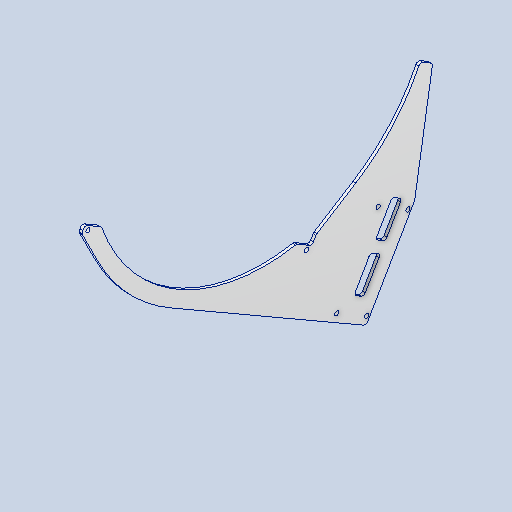
# Autodesk Inventor part: belt_liner_v2_Plate_6
Saved by Autodesk Inventor 2025.2 (Build 292293000, 293)
## iProperties
Created: 2025-01-06
Part Number: belt_liner_v2_Plate_6
Material: アルミニウム 6061
Document SubType Name: Modeling
Designer: haruy
Density: 2.7 g/cm^3
Appearance: アルミニウム - フラット
Author: haruy
Autodesk Inventor part; units mm, degrees
ref_plane "YZ Plane" through (0, 0, 0) normal (1, 0, 0) x (0, 1, 0)
ref_plane "XZ Plane" through (0, 0, 0) normal (0, 1, 0) x (-1, 0, 0)
ref_plane "XY Plane" through (0, 0, 0) normal (0, 0, 1) x (1, 0, 0)
derived "belt_liner_v2_Sketch_Base.ipt"
sketch "スケッチ1" plane through (300, 0, 0) normal (1, 0, 0) x (0, 1, 0)
  circle A0 centre (0, 0) radius 22.36
  circle A1 centre (742.400277, -428.625) radius 23.875 construction
  line L0 (0, 0) -> (0, -985.832038)
  line L1 (4.693429, 56.249257) -> (12.193429, 69.239638)
  line L2 (12.193429, 69.239638) -> (479.847147, -200.760362)
  line L3 (479.847147, -200.760362) -> (472.347147, -213.750743)
  line L4 (472.347147, -213.750743) -> (4.693429, 56.249257)
  line L5 (0, 0) -> (742.400277, -428.625)
  line L6 (-43.599071, -27.395807) -> (-51.099071, -40.386188)
  line L7 (-51.099071, -40.386188) -> (711.003284, -480.386188)
  line L8 (711.003284, -480.386188) -> (718.503284, -467.395807)
  line L9 (718.503284, -467.395807) -> (-43.599071, -27.395807)
  line L10 (-64.855825, 113.724045) -> (-64.855825, 113.724045)
  line L11 (4.693429, 56.249257) -> (0.351336, 58.756166)
  line L12 (0.351336, 58.756166) -> (-2.148664, 54.426038)
  line L13 (-2.148664, 54.426038) -> (2.193429, 51.91913)
  line L14 (2.193429, 51.91913) -> (4.693429, 56.249257)
  line L15 (472.347147, -213.750743) -> (374.172186, -157.069403)
  line L16 (0, -985.832038) -> (0, 0)
  circle A2 centre (0, 0) radius 12.5
  circle A3 centre (0, 0) radius 15
  line L17 (0, 0) -> (0, 0)
  circle A4 centre (0, 0) radius 24.06 construction
  line L18 (0, 0) -> (0, 0)
  line L19 (0, 0) -> (0, 0)
  line L20 (-43.599071, -27.395807) -> (-41.099071, -23.065679)
  line L21 (-41.099071, -23.065679) -> (28.918099, -63.490111)
  line L22 (32.480276, -71.320238) -> (-43.599071, -27.395807)
  line L23 (85.805588, 26.739638) -> (479.847147, -200.760362)
  line L24 (479.847147, -200.760362) -> (482.597147, -195.997222)
  circle A5 centre (742.400277, -428.625) radius 5
  line L25 (718.503284, -467.395807) -> (692.522522, -452.395807)
  line L26 (692.522522, -452.395807) -> (695.022522, -448.065679)
  line L27 (695.022522, -448.065679) -> (721.003284, -463.065679)
  line L28 (721.003284, -463.065679) -> (718.503284, -467.395807)
  circle A6 centre (738.07015, -426.125) radius 5.1
  line L29 (742.400277, -428.625) -> (511.038915, -295.048455)
  circle A7 centre (759.720785, -438.625) radius 5.1
  line L30 (740.62015, -421.70827) -> (762.270785, -434.20827)
  line L31 (735.52015, -430.54173) -> (757.170785, -443.04173)
  circle A8 centre (742.400277, -428.625) radius 22.175 construction
  line L32 (792.376136, -398.519566) -> (776.376136, -426.232379)
  line L33 (776.376136, -426.232379) -> (785.03639, -431.232379)
  line L34 (785.03639, -431.232379) -> (801.03639, -403.519566)
  line L35 (801.03639, -403.519566) -> (792.376136, -398.519566)
  circle A9 centre (738.07015, -426.125) radius 10.1 construction
  circle A10 centre (759.720785, -438.625) radius 10.1 construction
  line L36 (743.12015, -417.378143) -> (764.770785, -429.878143) construction
  line L37 (733.02015, -434.871857) -> (754.670785, -447.371857) construction
  line L38 (743.12015, -417.378143) -> (732.666299, -411.34261) construction
  line L39 (729.323294, -421.075) -> (734.373294, -412.328143) construction
  line L40 (764.770785, -429.878143) -> (773.093818, -434.683448) construction
  line L41 (773.093818, -434.683448) -> (773.43104, -434.878143)
  line L42 (0.351336, 58.756166) -> (-2.148664, 54.426038)
  line L43 (-2.148664, 54.426038) -> (100.487312, -4.83087)
  line L44 (100.487312, -4.83087) -> (102.987312, -0.500743)
  line L45 (102.987312, -0.500743) -> (0.351336, 58.756166)
  line L46 (-51.099071, -40.386188) -> (-51.099071, -619.920903)
  line L47 (754.670785, -447.371857) -> (764.770785, -429.878143)
  line L48 (764.770785, -429.878143) -> (773.43104, -434.878143)
  line L49 (773.43104, -434.878143) -> (763.33104, -452.371857)
  line L50 (763.33104, -452.371857) -> (754.670785, -447.371857) construction
  line L51 (479.847147, -200.760362) -> (472.347147, -213.750743)
  line L52 (472.347147, -213.750743) -> (896.699557, -458.750721)
  line L53 (896.699557, -458.750721) -> (904.199557, -445.76034)
  line L54 (904.199557, -445.76034) -> (479.847147, -200.760362)
  line L55 (-12.152186, -2.928204) -> (-38.10869, -47.886188)
  line L56 (-12.152186, -2.928204) -> (25.18381, 61.739638)
  circle A11 centre (38.084445, 34.084194) radius 1.5
  circle A12 centre (59.73508, 21.584194) radius 1.5
  circle A13 centre (711.09303, -460.230743) radius 1.5
  circle A14 centre (0, 0) radius 60
  line L57 (54.694812, -84.145807) -> (57.194812, -79.815679)
  line L58 (100.487312, -4.83087) -> (57.194812, -79.815679)
  circle A15 centre (81.385715, 9.084194) radius 1.5
  circle A16 centre (742.400277, -428.625) radius 6 construction
  circle A17 centre (0, 0) radius 24.06 construction
  circle A18 centre (0, 0) radius 24.06
  circle A19 centre (742.400277, -428.625) radius 24.06
  line L59 (754.430277, -407.788429) -> (12.03, 20.836571)
  circle A20 centre (725.859192, -419.075) radius 4
  circle A21 centre (725.859192, -419.075) radius 1.5
  circle A22 centre (742.400277, -428.625) radius 18.525 construction
  circle A23 centre (748.98688, -417.41667) radius 4
  line L60 (737.43688, -437.421857) -> (742.48688, -428.675)
  circle A24 centre (748.98688, -417.41667) radius 1.5
  line L61 (734.373294, -412.328143) -> (737.823294, -406.352568) construction
  line L62 (737.823294, -406.352568) -> (776.88104, -428.902568)
  line L63 (773.43104, -434.878143) -> (776.88104, -428.902568)
  line L64 (737.823294, -406.352568) -> (723.650341, -415.740187)
  line L65 (720.823294, -435.797432) -> (759.88104, -458.347432)
  line L66 (720.823294, -435.797432) -> (721.866734, -418.829485)
  line L67 (763.33104, -452.371857) -> (759.88104, -458.347432)
  circle A25 centre (735.98688, -439.93333) radius 4
  circle A26 centre (735.98688, -439.93333) radius 1.5
  circle A27 centre (300.529907, 58.653068) radius 120
  line L68 (24.788304, 15.779962) -> (16.12805, 20.779962) construction
  line L69 (896.699557, -458.750721) -> (870.718795, -443.750721)
  line L70 (870.718795, -443.750721) -> (868.218795, -448.080848)
  line L71 (868.218795, -448.080848) -> (894.199557, -463.080848)
  line L72 (894.199557, -463.080848) -> (896.699557, -458.750721)
  circle A28 centre (886.789303, -455.915785) radius 1.5
  line L73 (100.487312, -4.83087) -> (102.987312, -0.500743)
  line L74 (102.987312, -0.500743) -> (112.946604, -6.250743)
  line L75 (112.946604, -6.250743) -> (110.446604, -10.58087)
  line L76 (110.446604, -10.58087) -> (100.487312, -4.83087)
  circle A29 centre (878.129049, -450.915785) radius 1.5
  circle A30 centre (702.432776, -455.230743) radius 1.5
  line L77 (28.918099, -63.490111) -> (57.194812, -79.815679)
  line L78 (479.847147, -200.760362) -> (482.597147, -195.997222)
  line L79 (121.446604, 8.471689) -> (179.903319, -25.278311)
  line L80 (179.903319, -25.278311) -> (182.403319, -20.948184)
  line L81 (182.403319, -20.948184) -> (123.946604, 12.801816)
  line L82 (123.946604, 12.801816) -> (121.446604, 8.471689)
  circle A31 centre (135.905896, 10.515918) radius 4
  circle A32 centre (135.905896, 10.515918) radius 11
  circle A33 centre (161.886659, -4.484082) radius 4
  circle A34 centre (161.886659, -4.484082) radius 11
  line L83 (131.869998, -4.474463) -> (128.369998, -10.536641)
  line L84 (128.369998, -10.536641) -> (147.422557, -21.536641)
  line L85 (147.422557, -21.536641) -> (150.922557, -15.474463)
  line L86 (150.922557, -15.474463) -> (131.869998, -4.474463)
  line L87 (141.396277, -9.974463) -> (137.896277, -16.036641)
  line L88 (157.85076, -19.474463) -> (154.35076, -25.536641)
  line L89 (154.35076, -25.536641) -> (173.403319, -36.536641)
  line L90 (173.403319, -36.536641) -> (176.903319, -30.474463)
  line L91 (176.903319, -30.474463) -> (157.85076, -19.474463)
  line L92 (167.37704, -24.974463) -> (163.87704, -31.036641)
  line L93 (8.443429, 62.744448) -> (900.449557, -452.255531)
  line L94 (170.403319, -41.732794) -> (167.903319, -46.062921)
  line L95 (111.946604, -7.982794) -> (170.403319, -41.732794)
  line L96 (167.903319, -46.062921) -> (109.446604, -12.312921)
  line L97 (109.446604, -12.312921) -> (111.946604, -7.982794)
  circle A35 centre (117.405896, -21.527022) radius 11
  circle A36 centre (117.405896, -21.527022) radius 4
  circle A37 centre (143.386659, -36.527022) radius 11
  circle A38 centre (143.386659, -36.527022) radius 4
  line L98 (140.932176, -2.778311) -> (147.860379, -6.778311)
  line L99 (147.860379, -6.778311) -> (138.360379, -23.232794)
  line L100 (138.360379, -23.232794) -> (131.432176, -19.232794)
  line L101 (131.432176, -19.232794) -> (140.932176, -2.778311)
  line L102 (166.912938, -17.778311) -> (173.841141, -21.778311)
  line L103 (173.841141, -21.778311) -> (164.341141, -38.232794)
  line L104 (164.341141, -38.232794) -> (157.412938, -34.232794)
  line L105 (157.412938, -34.232794) -> (166.912938, -17.778311)
  line L106 (109.446604, -12.312921) -> (96.946604, -33.963556)
  line L107 (96.946604, -33.963556) -> (105.606858, -38.963556)
  line L108 (105.606858, -38.963556) -> (118.106858, -17.312921)
  line L109 (118.106858, -17.312921) -> (109.446604, -12.312921)
  line L110 (109.446604, -12.312921) -> (144.953646, -32.812921)
  line L111 (144.953646, -32.812921) -> (140.953646, -39.741124)
  line L112 (140.953646, -39.741124) -> (105.446604, -19.241124)
  line L113 (105.446604, -19.241124) -> (109.446604, -12.312921)
  line L114 (128.932176, -23.562921) -> (135.860379, -27.562921)
  line L115 (135.860379, -27.562921) -> (134.360379, -30.160997)
  line L116 (134.360379, -30.160997) -> (127.432176, -26.160997)
  line L117 (127.432176, -26.160997) -> (128.932176, -23.562921)
  circle A39 centre (-7.708055, -45.230743) radius 1.25
  circle A40 centre (13.94258, -57.730743) radius 1.25
  circle A41 centre (35.593215, -70.230743) radius 1.25
  circle A42 centre (300.529907, 58.653068) radius 130
  line L118 (300.529907, 58.653068) -> (196.606858, 118.653068)
  line L119 (300.529907, 58.653068) -> (184.618808, 27.594782)
  line L120 (300.529907, 58.653068) -> (269.471621, 174.564167)
  line L121 (272.471621, 179.760319) -> (181.618808, 22.39863)
  line L122 (181.618808, 22.39863) -> (176.422655, 25.39863)
  line L123 (176.422655, 25.39863) -> (267.275469, 182.760319)
  line L124 (267.275469, 182.760319) -> (272.471621, 179.760319)
  line L125 (300.529907, 58.653068) -> (235.529907, -53.930235)
  line L126 (791.376136, -400.251617) -> (788.876136, -404.581744)
  line L127 (788.876136, -404.581744) -> (847.332851, -438.331744)
  line L128 (847.332851, -438.331744) -> (849.832851, -434.001617)
  line L129 (849.832851, -434.001617) -> (791.376136, -400.251617)
  line L130 (849.832851, -434.001617) -> (847.332851, -438.331744)
  line L131 (847.332851, -438.331744) -> (867.218795, -449.812899)
  line L132 (867.218795, -449.812899) -> (869.718795, -445.482772)
  line L133 (869.718795, -445.482772) -> (849.832851, -434.001617)
  line L134 (737.823294, -406.352568) -> (868.218795, -448.080848)
  circle A43 centre (742.400277, -428.625) radius 34.06
  line L135 (859.244569, -445.208978) -> (862.744569, -439.1468)
  circle A44 centre (742.48688, -428.675) radius 8.5
  line L136 (253.202227, 236.679121) -> (109.446604, -12.312921)
  line L137 (249.398857, -49.908508) -> (244.382754, -58.596654)
  line L138 (244.382754, -58.596654) -> (167.903319, -46.062921)
  line L139 (181.618808, 22.39863) -> (198.870869, -5.107736)
  line L140 (267.275469, 182.760319) -> (268.340368, 184.604779)
  circle A45 centre (127.026731, 8.136752) radius 1.5
  circle A46 centre (176.823192, -20.613248) radius 1.5
  circle A47 centre (115.026731, -12.647857) radius 1.5
  circle A48 centre (164.823192, -41.397857) radius 1.5
  line L141 (131.686985, -3.791451) -> (127.686985, -10.719654)
  line L142 (127.686985, -10.719654) -> (147.60557, -22.219654)
  line L143 (147.60557, -22.219654) -> (151.60557, -15.291451)
  line L144 (151.60557, -15.291451) -> (131.686985, -3.791451)
  line L145 (157.667747, -18.791451) -> (153.667747, -25.719654)
  line L146 (153.667747, -25.719654) -> (173.586332, -37.219654)
  line L147 (173.586332, -37.219654) -> (177.586332, -30.291451)
  line L148 (177.586332, -30.291451) -> (157.667747, -18.791451)
  line L149 (176.422655, 25.39863) -> (179.422655, 30.594782)
  line L150 (179.422655, 30.594782) -> (175.092528, 33.094782)
  line L151 (175.092528, 33.094782) -> (172.092528, 27.89863)
  line L152 (172.092528, 27.89863) -> (176.422655, 25.39863)
  line L153 (267.275469, 182.760319) -> (264.275469, 177.564167)
  line L154 (264.275469, 177.564167) -> (259.945342, 180.064167)
  line L155 (259.945342, 180.064167) -> (262.945342, 185.260319)
  line L156 (262.945342, 185.260319) -> (267.275469, 182.760319)
  circle A49 centre (263.610405, 181.412243) radius 1.5
  line L157 (268.340368, 184.604779) -> (262.945342, 185.260319)
  line L158 (262.945342, 185.260319) -> (242.144586, 174.804496)
  circle A50 centre (175.757592, 29.246706) radius 1.5
  line L159 (894.199557, -463.080848) -> (718.503284, -467.395807)
  line L160 (695.022522, -448.065679) -> (722.856178, -416.43267)
  line L161 (870.718795, -443.750721) -> (868.218795, -448.080848)
  line L162 (868.218795, -448.080848) -> (861.290592, -444.080848)
  line L163 (861.290592, -444.080848) -> (863.790592, -439.750721)
  line L164 (863.790592, -439.750721) -> (870.718795, -443.750721)
  line L165 (-33.353881, -27.640997) -> (-48.353881, -27.640997)
  line L166 (-48.353881, -27.640997) -> (-48.353881, -280.140997)
  line L167 (-48.353881, -280.140997) -> (-33.353881, -280.140997)
  line L168 (-33.353881, -280.140997) -> (-33.353881, -27.640997)
  line L169 (331.646119, -265.140997) -> (-48.353881, -265.140997)
  line L170 (-48.353881, -265.140997) -> (-48.353881, -280.140997)
  line L171 (-48.353881, -280.140997) -> (331.646119, -280.140997)
  line L172 (331.646119, -280.140997) -> (331.646119, -265.140997)
  line L173 (-20.788182, -57.886188) -> (-13.288182, -44.895807)
  line L174 (5.19258, -72.886188) -> (12.69258, -59.895807)
  line L175 (-48.353881, -74.640997) -> (-71.353881, -74.640997)
  line L176 (-71.353881, -74.640997) -> (-71.353881, -134.640997)
  line L177 (-71.353881, -134.640997) -> (-48.353881, -134.640997)
  line L178 (-48.353881, -134.640997) -> (-48.353881, -74.640997)
  line L179 (-48.353881, -94.640997) -> (-93.353881, -94.640997)
  line L180 (-93.353881, -94.640997) -> (-93.353881, -114.640997)
  line L181 (-93.353881, -114.640997) -> (-48.353881, -114.640997)
  line L182 (-48.353881, -114.640997) -> (-48.353881, -94.640997)
  line L183 (-33.353881, -74.640997) -> (-48.353881, -74.640997)
  line L184 (-93.353881, -104.640997) -> (-48.353881, -104.640997)
  line L185 (-57.353881, -244.640997) -> (-62.353881, -244.640997)
  line L186 (-62.353881, -244.640997) -> (-62.353881, -254.640997)
  line L187 (-62.353881, -254.640997) -> (-57.353881, -254.640997)
  line L188 (-57.353881, -254.640997) -> (-57.353881, -244.640997)
  line L189 (-48.353881, -236.142687) -> (-53.353881, -236.142687)
  line L190 (-53.353881, -236.142687) -> (-53.353881, -262.050693)
  line L191 (-53.353881, -262.050693) -> (-48.353881, -262.050693)
  line L192 (-48.353881, -262.050693) -> (-48.353881, -236.142687)
  line L193 (-50.853881, -236.142687) -> (-50.853881, -262.050693)
  line L194 (301.646119, -265.140997) -> (301.646119, -280.140997)
  line L195 (331.646119, -280.140997) -> (364.16844, -280.140997)
  line L196 (364.16844, -280.140997) -> (371.66844, -267.150616)
  line L197 (331.646119, -265.140997) -> (338.187678, -265.140997)
  line L198 (338.187678, -265.140997) -> (345.687678, -252.150616)
  line L199 (-62.353881, -249.640997) -> (-57.353881, -249.640997)
  line L200 (-89.353881, 250.218666) -> (-109.353881, 250.218666)
  line L201 (-109.353881, 250.218666) -> (-109.353881, -699.60028)
  line L202 (-109.353881, -699.60028) -> (-89.353881, -699.60028)
  line L203 (-89.353881, -699.60028) -> (-89.353881, 250.218666)
  line L204 (263.610405, 181.412243) -> (-89.353881, 181.412243)
  line L205 (-26.7774, -265.289513) -> (-29.28918, -274.968922)
  line L206 (-29.28918, -274.968922) -> (688.535788, -461.242481)
  line L207 (688.535788, -461.242481) -> (691.047567, -451.563072)
  line L208 (691.047567, -451.563072) -> (-26.7774, -265.289513)
  line L209 (-48.353881, -157.96965) -> (-50.353881, -157.96965)
  line L210 (-50.353881, -157.96965) -> (-50.353881, -198.398984)
  line L211 (-50.353881, -198.398984) -> (-48.353881, -198.398984)
  line L212 (-48.353881, -198.398984) -> (-48.353881, -157.96965)
  line L213 (-48.353881, -162.0415) -> (22.746119, -162.0415)
  line L214 (22.746119, -162.0415) -> (22.746119, -204.0415)
  line L215 (22.746119, -204.0415) -> (-48.353881, -204.0415)
  line L216 (-48.353881, -204.0415) -> (-48.353881, -162.0415)
  line L217 (-48.353881, -165.433743) -> (-51.353881, -165.433743)
  line L218 (-51.353881, -165.433743) -> (-51.353881, -191.433743)
  line L219 (-51.353881, -191.433743) -> (-48.353881, -191.433743)
  line L220 (-48.353881, -191.433743) -> (-48.353881, -165.433743)
  line L221 (-51.353881, -177.494923) -> (-75.653881, -177.494923)
  line L222 (-75.653881, -177.494923) -> (-75.653881, -187.494923)
  line L223 (-75.653881, -187.494923) -> (-51.353881, -187.494923)
  line L224 (-51.353881, -187.494923) -> (-51.353881, -177.494923)
  line L225 (-56.353881, -167.251042) -> (-66.353881, -167.251042)
  line L226 (-66.353881, -167.251042) -> (-66.353881, -197.251042)
  line L227 (-66.353881, -197.251042) -> (-56.353881, -197.251042)
  line L228 (-56.353881, -197.251042) -> (-56.353881, -167.251042)
  line L229 (-66.353881, -156.211182) -> (-72.353881, -156.211182)
  line L230 (-72.353881, -156.211182) -> (-72.353881, -222.344302)
  line L231 (-72.353881, -222.344302) -> (-66.353881, -222.344302)
  line L232 (-66.353881, -222.344302) -> (-66.353881, -156.211182)
  circle A51 centre (986.855039, -337.596932) radius 120
  line L233 (54.694812, -84.145807) -> (57.194812, -79.815679)
  line L234 (57.194812, -79.815679) -> (67.154104, -85.565679)
  line L235 (67.154104, -85.565679) -> (64.654104, -89.895807)
  line L236 (64.654104, -89.895807) -> (54.694812, -84.145807)
  line L237 (-43.599071, -27.395807) -> (2.193429, 51.91913)
  line L238 (-19.452821, 14.426725) -> (142.076282, -78.832146)
  circle A52 centre (74.61885, -7.551639) radius 15
  line L239 (64.654104, -89.895807) -> (112.946604, -6.250743)
  circle A53 centre (74.61885, -7.551639) radius 22
  circle A54 centre (67.149719, -35.573275) radius 5
  circle A55 centre (103.616477, -12.410997) radius 5
  circle A56 centre (65.323977, -78.735552) radius 5
  circle A57 centre (11.759787, -74.072312) radius 15
  circle A58 centre (48.161986, -57.492809) radius 15
  circle A59 centre (48.161986, -57.492809) radius 22
  circle A60 centre (0, 0) radius 24.06
  line L240 (854.261054, -442.331744) -> (857.761054, -436.269566) construction
  line L241 (861.290592, -444.080848) -> (863.790592, -439.750721)
  line L242 (863.790592, -439.750721) -> (857.728414, -436.250721)
  line L243 (857.728414, -436.250721) -> (855.228414, -440.580848)
  line L244 (855.228414, -440.580848) -> (861.290592, -444.080848)
  line L245 (849.832851, -434.001617) -> (864.427288, -408.723309)
  line L246 (859.332851, -417.547134) -> (861.832851, -413.217007)
  line L247 (861.832851, -413.217007) -> (842.253241, -401.912714)
  line L248 (842.253241, -401.912714) -> (839.753241, -406.242841)
  line L249 (839.753241, -406.242841) -> (859.332851, -417.547134)
  line L250 (913.524875, -454.608416) -> (917.855002, -457.108416)
  line L251 (917.855002, -457.108416) -> (928.855002, -438.055858)
  line L252 (928.855002, -438.055858) -> (924.524875, -435.555858)
  line L253 (924.524875, -435.555858) -> (913.524875, -454.608416)
  line L254 (916.024875, -450.278289) -> (922.024875, -439.885985)
  line L255 (922.024875, -439.885985) -> (909.900519, -432.885985)
  line L256 (909.900519, -432.885985) -> (903.900519, -443.278289)
  line L257 (903.900519, -443.278289) -> (916.024875, -450.278289)
  line L258 (905.400519, -440.680213) -> (908.400519, -435.484061)
  line L259 (908.400519, -435.484061) -> (863.832851, -409.752905)
  line L260 (863.832851, -409.752905) -> (860.832851, -414.949058)
  line L261 (860.832851, -414.949058) -> (905.400519, -440.680213)
  line L262 (878.08963, -417.984061) -> (875.08963, -423.180213)
  line L263 (897.271354, -441.76034) -> (902.900519, -445.01034)
  line L264 (924.524875, -435.555858) -> (907.524875, -465.000721)
  line L265 (907.524875, -465.000721) -> (903.194748, -462.500721)
  line L266 (903.194748, -462.500721) -> (920.194748, -433.055858)
  line L267 (920.194748, -433.055858) -> (924.524875, -435.555858)
  line L268 (896.699557, -458.750721) -> (907.524875, -465.000721)
  line L269 (907.524875, -465.000721) -> (905.024875, -469.330848)
  line L270 (905.024875, -469.330848) -> (894.199557, -463.080848)
  line L271 (894.199557, -463.080848) -> (896.699557, -458.750721)
  point P0 (732.666299, -411.34261)
  point P1 (-0.898664, 56.591102)
  point P2 (182.651593, 36.187467)
  point P3 (261.046531, 171.971482)
  point P4 (187.946604, 123.653068)
  point P5 (242.144586, 174.804496)
  point P6 (-30.60869, -34.895807)
  point P7 (-40.853881, -37.640997)
  point P8 (-40.853881, -272.640997)
  point P9 (321.646119, -272.640997)
  point P10 (311.646119, -272.640997)
  point P11 (351.022615, -263.890997)
  point P12 (359.682869, -268.890997)
  point P13 (-18.353881, -272.640997)
  point P14 (680.112268, -453.890997)
  dimension "d3" = 0.5
  dimension "d4" = 0.5
  measures "d3" distance between parallel lines of L86 L144
  measures "d4" distance between parallel lines of L91 L148
extrude "押し出し1" add sketch "スケッチ1" against normal blind 2 contours L136 L2 L101 L144 L141 L93 | L93 L141 L142 L101 L4 L136 | L141 L144 L101 L86 L83 L93 | L93 L83 L84 L101 L142 L141 | L136 L79 A32 L2 | L4 A35 L95 L75 | L75 L95 A35 L96 L97 | L93 L101 L84 L83 | L83 L86 L101 L93 | A32 L79 L101 L2 | A32 L79 | L82 L81 A32 L79 | L4 L101 L95 A35 | A35 L95 | L101 L86 L87 L93 | L93 L87 L84 L101 | L144 L99 L86 L101 | L101 L2 L99 L144 | L142 L99 L4 L101 | L101 L84 L99 L142 | L101 L79 L99 L2 | A32 L81 L79 | A32 L81 A34 L79 | L136 A42 L151 L152 L138 L2 L103 L79 L80 L81 A34 A32 | L4 L99 L95 L101 | A35 L96 L95 | L95 A37 L96 A35 | L93 L99 L84 L87 | L87 L86 L99 L93 | L144 L143 L93 L85 L86 L99 | L99 L2 L105 L148 L145 L93 L143 L144 | L142 L143 L93 L145 L146 L105 L4 L99 | L99 L84 L85 L93 L143 L142 | L99 L79 A34 L2 | A31 | A32 L81 | A42 L204 L155 L154 L123 A27 L150 L151 | L4 A37 L95 L99 | L99 L86 L85 L93 | L93 L85 L84 L99 | A34 L79 L105 L2 | A34 L79 | A33 | A34 L81 | L81 A34 L79 | L151 L150 L123 L152 A42 | A42 L152 L151 | L4 L105 L95 A37 | A37 L95 | A37 L95 L96 | A37 L95 L94 L96 | L105 L79 L103 L2 | L2 L103 L148 L105 | A34 L81 L80 L79 | A42 L155 L204 | L152 L122 L139 A27 L125 A42 | L105 L146 L103 L4 | L4 L103 L95 L105 | L94 L95 L103 L4 L138 | L145 L148 L105 L91 L88 L93 | L93 L88 L89 L105 L146 L145 | L2 L138 L93 L147 L148 L103 | L148 L103 L91 L105 | A42 L156 L123 L154 L155 | L125 A27 L137 A42 | L103 L146 L147 L93 L138 L4 | L105 L89 L103 L146 | L93 L105 L89 L88 | L88 L91 L105 L93 | L148 L147 L93 L90 L91 L103 | L91 L92 L93 L105 | A42 L140 L156 | L103 L89 L90 L93 L147 L146 | L105 L93 L92 L89 | L103 L93 L92 L91 | L91 L90 L93 L103 | L103 L93 L90 L89 | L89 L92 L93 L103 | A49 | A50
extrude "押し出し2" cut sketch "スケッチ1" against normal blind 10 contours L141 L144 L101 L86 L83 L93 | L93 L83 L84 L101 L142 L141 | L93 L101 L84 L83 | L83 L86 L101 L93 | L101 L86 L87 L93 | L93 L87 L84 L101 | L144 L99 L86 L101 | L101 L84 L99 L142 | L93 L99 L84 L87 | L87 L86 L99 L93 | L144 L143 L93 L85 L86 L99 | L99 L84 L85 L93 L143 L142 | L99 L86 L85 L93 | L93 L85 L84 L99 | L145 L148 L105 L91 L88 L93 | L93 L88 L89 L105 L146 L145 | L148 L103 L91 L105 | L105 L89 L103 L146 | L93 L105 L89 L88 | L88 L91 L105 L93 | L148 L147 L93 L90 L91 L103 | L91 L92 L93 L105 | L103 L89 L90 L93 L147 L146 | L105 L93 L92 L89 | L103 L93 L92 L91 | L91 L90 L93 L103 | L103 L93 L90 L89 | L89 L92 L93 L103
extrude "押し出し3" add sketch "スケッチ1" against normal blind 2 contours L158 L204 A42 | L204 L158 L155 A42 | L155 L156 A42 | L157 A42 L156
extrude "押し出し4" cut sketch "スケッチ1" against normal blind 2 contours A49 | A50
fillet "フィレット1" radius 2 18 edges at (299, 109.4466, -12.3129) (299, 167.9033, -46.0629) (299, 244.3828, -58.5967) (299, 249.3989, -49.9085) (299, 176.4227, 25.3986) (299, 181.6188, 22.3986) (299, 182.6516, 36.1875) (299, 261.0465, 171.9715) (299, 268.3404, 184.6048) (299, 262.9453, 185.2603) (299, 151.6056, -15.2915) (299, 131.687, -3.7915) (299, 127.687, -10.7197) (299, 147.6056, -22.2197) (299, 153.6677, -25.7197) (299, 157.6677, -18.7915) (299, 177.5863, -30.2915) (299, 173.5863, -37.2197)
